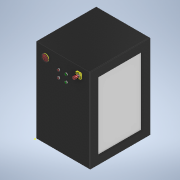
# Autodesk Inventor part: Tablero Maya
Saved by Autodesk Inventor 2020 (Build 240168000, 168)
## iProperties
Created: 2019-10-05
Part Number: Tablero Maya
Material: Genérico
Document SubType Name: Modeling
Designer: dasa1
Density: 1 g/cm^3
Appearance: Valor por defecto
Author: dasa1
Autodesk Inventor part; units mm, degrees
ref_plane "YZ Plane" through (0, 0, 0) normal (1, 0, 0) x (0, 1, 0)
ref_plane "XZ Plane" through (0, 0, 0) normal (0, 1, 0) x (-1, 0, 0)
ref_plane "XY Plane" through (0, 0, 0) normal (0, 0, 1) x (1, 0, 0)
sketch "Boceto1" plane through (0, 0, 0) normal (0, 1, 0) x (-1, 0, 0)
  line L0 (0, 0) -> (-530, 0)
  line L1 (-530, 0) -> (-530, -600)
  line L2 (-530, -600) -> (0, -600)
  line L3 (0, -600) -> (0, 0)
  dimension "d0" = 530
  dimension "d1" = 600
  constraints: 8 end point, 2 parallel, 1 horizontal, 1 perpendicular
  measures "d0" distance of L2.end L1.end
  measures "d1" distance of L1.end L0.end
extrude "Extrusión1" add sketch "Boceto1" along normal blind 840
sketch "Boceto2" plane through (530, 0, 0) normal (1, 0, 0) x (0, 0, -1)
  line L0 (0, 0) -> (0, 840) projected
  line L1 (0, 840) -> (10, 840)
  line L2 (10, 840) -> (10, 830)
  line L3 (10, 830) -> (0, 830)
  line L4 (0, 830) -> (0, 840)
  line L5 (10, 830) -> (590, 830)
  line L6 (590, 830) -> (590, 10)
  line L7 (590, 10) -> (10, 10)
  line L8 (10, 10) -> (10, 830)
  dimension "d4" = 10
  dimension "d5" = 10
  dimension "d6" = 580
  dimension "d7" = 820
  constraints: 16 end point, 4 parallel, 2 horizontal, 2 perpendicular
  measures "d4" distance of L2.end L3.end
  measures "d5" distance of L1.end L2.end
  measures "d6" distance of L6.end L7.end
  measures "d7" distance of L5.end L6.end
extrude "Extrusión2" cut sketch "Boceto2" against normal blind 520 contours L5 L6 L7 L8
sketch "Boceto3" plane through (0, 0, 0) normal (0, 0, 1) x (1, 0, 0)
  line L0 (530, 830) -> (10, 830) projected
  line L1 (10, 830) -> (520, 830) construction
  line L2 (520, 830) -> (520, 580) construction
  line L3 (520, 580) -> (10, 580) construction
  line L4 (10, 580) -> (10, 830) construction
  line L5 (265, 830) -> (265, 580) construction
  line L6 (265, 580) -> (265, 640)
  line L7 (265, 640) -> (290, 640) construction
  line L8 (265, 640) -> (240, 640) construction
  line L9 (290, 640) -> (302.5, 640) construction
  line L10 (240, 640) -> (227.5, 640) construction
  circle A0 centre (302.5, 640) radius 12.5
  circle A1 centre (227.5, 640) radius 12.5
  line L11 (227.5, 640) -> (227.5, 710) construction
  line L12 (302.5, 640) -> (302.5, 710) construction
  circle A2 centre (227.5, 710) radius 12.5
  circle A3 centre (302.5, 710) radius 12.5
  line L13 (10, 830) -> (10, 10) construction
  line L14 (10, 830) -> (10, 705) construction
  point P0 (0, 0)
  dimension "d10" = 510
  dimension "d11" = 250
  dimension "d12" = 255
  dimension "d13" = 0
  dimension "d14" = 60
  dimension "d15" = 25
  dimension "d16" = 25
  dimension "d17" = 12.5
  dimension "d18" = 12.5
  dimension "d19" = 70
  dimension "d20" = 70
  dimension "d21" = 25
  dimension "d22" = 25
  dimension "d23" = 125
  constraints: 26 end point, 4 coincident, 4 horizontal, 3 perpendicular, 2 centre point, 2 horizontal alignment, 2 parallel, 2 point on line, 2 vertical, 1 midpoint, 4 other
  measures "d10" distance of L2.end L3.end
  measures "d11" distance of L1.end L2.end
  measures "d12" distance between parallel lines of L5 L2
  measures "d13" distance from line of L5.start L0
  measures "d14" distance of L5.end L6.end
  measures "d15" distance of L6.end L7.end
  measures "d16" distance of L6.end L8.end
  measures "d17" distance of L7.end L9.end
  measures "d18" distance of L8.end L10.end
  measures "d19" distance of L11.start L11.end
  measures "d20" distance of L12.start L12.end
  measures "d21" diameter of A2
  measures "d22" diameter of A3
  measures "d23" distance of L0.end L14.end
extrude "Extrusión3" add sketch "Boceto3" along normal blind 10
sketch "Boceto4" plane through (302.5, 710, 10) normal (0, 0, 1) x (1, 0, 0)
  circle A0 centre (0, 0) radius 11.5
  circle A1 centre (-75, 0) radius 12.5 projected
  circle A2 centre (-75, 0) radius 11.5
  circle A3 centre (-75, 0) radius 12.5
  circle A4 centre (0, -70) radius 12.5 projected
  circle A5 centre (-75, 0) radius 12.5 projected
  circle A6 centre (-75, -70) radius 12.5 projected
  circle A7 centre (0, 0) radius 12.5 projected
  line L0 (-302.5, -710) -> (227.5, -710) projected
  line L1 (227.5, -710) -> (227.5, 130) projected
  line L2 (-302.5, 130) -> (227.5, 130) projected
  line L3 (-302.5, -710) -> (-302.5, 130) projected
  line L4 (-302.5, -710) -> (-302.5, 130) projected
  line L5 (0, 0) -> (-302.5, 0)
  line L6 (-302.5, 0) -> (-302.5, -710)
  line L7 (-302.5, -710) -> (0, -710)
  line L8 (0, -710) -> (0, 0)
  dimension "d26" = 23
  dimension "d27" = 23
  dimension "d29" = 75
  dimension "d30" = 710
  dimension "d31" = 302.5
  constraints: 8 end point, 3 centre point, 2 coincident, 2 parallel, 1 concentric, 1 horizontal, 1 perpendicular
  measures "d26" diameter of A0
  measures "d27" diameter of A2
  measures "d29" distance of A1.centre A0.centre
  measures "d30" distance of L7.end A0.centre
  measures "d31" distance of L0.start L7.end
extrude "Extrusión4" cut sketch "Boceto4" against normal blind 2 contours A0 L8 L5 | L5 L8 A0 | L5 A2 | A2 L5
fillet "Empalme1" radius 3 2 edges at (215, 640, 10) (290, 640, 10)
sketch "Boceto5" plane through (0, 0, 0) normal (0, 0, 1) x (1, 0, 0)
  circle A0 centre (302.5, 640) radius 12.5 projected
  circle A1 centre (227.5, 710) radius 12.5 projected
  circle A2 centre (227.5, 640) radius 12.5 projected
  circle A3 centre (302.5, 710) radius 12.5 projected
  line L0 (0, 0) -> (530, 0) projected
  line L1 (530, 0) -> (530, 840) projected
  line L2 (0, 840) -> (530, 840) projected
  line L3 (0, 0) -> (0, 840) projected
  line L4 (530, 830) -> (10, 830) construction
  line L5 (10, 830) -> (520, 830) construction
  line L6 (520, 830) -> (520, 630) construction
  line L7 (520, 630) -> (10, 630) construction
  line L8 (10, 630) -> (10, 830) construction
  line L9 (520, 630) -> (435, 630) construction
  line L10 (435, 630) -> (435, 770) construction
  line L11 (10, 630) -> (75, 630) construction
  line L12 (75, 630) -> (75, 770) construction
  line L13 (435, 770) -> (435, 795) construction
  line L14 (435, 795) -> (410, 795) construction
  line L15 (410, 795) -> (460, 795)
  line L16 (460, 795) -> (460, 745)
  line L17 (460, 745) -> (410, 745)
  line L18 (410, 745) -> (410, 795)
  dimension "d35" = 510
  dimension "d36" = 200
  dimension "d37" = 85
  dimension "d38" = 140
  dimension "d39" = 65
  dimension "d40" = 140
  dimension "d41" = 25
  dimension "d42" = 25
  dimension "d43" = 50
  dimension "d44" = 50
  constraints: 28 end point, 5 perpendicular, 4 parallel, 2 horizontal, 2 point on line, 1 vertical
  measures "d35" distance of L6.end L7.end
  measures "d36" distance of L5.end L6.end
  measures "d37" distance of L6.end L9.end
  measures "d38" distance of L9.end L10.end
  measures "d39" distance of L7.end L11.end
  measures "d40" distance of L11.end L12.end
  measures "d41" distance of L13.end L14.end
  measures "d42" distance of L10.end L13.end
  measures "d43" distance of L16.end L17.end
  measures "d44" distance of L15.end L16.end
extrude "Extrusión5" add sketch "Boceto5" along normal blind 15 contours L15 L16 L17 L18
sketch "Boceto7" plane through (0, 0, 15) normal (0, 0, 1) x (1, 0, 0)
  line L0 (410, 745) -> (460, 745) construction
  line L1 (460, 745) -> (460, 795) construction
  line L2 (460, 795) -> (410, 795) construction
  line L3 (410, 795) -> (410, 745) construction
  line L4 (460, 745) -> (410, 745) construction
  line L5 (410, 745) -> (435, 745) construction
  line L6 (435, 745) -> (435, 770) construction
  line L7 (435, 770) -> (410, 770) construction
  line L8 (410, 770) -> (410, 745) construction
  point P0 (0, 0)
  dimension "d53" = 25
  dimension "d54" = 25
  constraints: 8 end point, 2 parallel, 1 horizontal, 1 perpendicular
  measures "d53" distance of L7.end L6.end
  measures "d54" distance of L6.end L5.end
ref_plane "Plano de trabajo1" through (435, 770, 15) normal (-1, 0, 0) x (0, -1, 0)
sketch "Boceto8" plane through (435, 770, 15) normal (-1, 0, 0) x (0, -1, 0)
  line L0 (-25, 0) -> (25, 0) construction
  line L1 (0, 0) -> (0, 50)
  line L2 (0, 0) -> (50, 0) construction
  line L3 (0, 50) -> (-15, 50)
  line L4 (0, 50) -> (15, 50) construction
  line L5 (-15, 50) -> (-15, 40)
  line L6 (0, 0) -> (-10, 0)
  line L7 (-10, 0) -> (-15, 40)
  point P0 (770, -15)
  dimension "d55" = 50
  dimension "d56" = 90
  dimension "d57" = 15
  dimension "d58" = 180
  dimension "d59" = 10
  dimension "d60" = 10
  constraints: 14 end point, 3 horizontal, 2 equal length, 1 midpoint, 1 perpendicular, 1 point on line, 1 vertical
  measures "d55" distance of L1.start L1.end
  measures "d56" angle of L2 L1
  measures "d57" distance of L1.end L3.end
  measures "d58" angle of L3 L4
  measures "d59" distance of L3.end L5.end
  measures "d60" distance of L1.start L6.end
revolve "Revolución1" add sketch "Boceto8" angle 360 about axis through (435, 770, 15) along (0, 0, 1)
fillet "Empalme3" radius 5 1 edges at (435, 755, 65)
fillet "Empalme4" radius 5 1 edges at (435, 760, 15)
sketch "Boceto9" plane through (0, 0, 0) normal (0, 0, 1) x (1, 0, 0)
  line L0 (530, 830) -> (10, 830) construction
  line L1 (10, 830) -> (10, 10) construction
  line L2 (10, 830) -> (520, 830) construction
  line L3 (520, 830) -> (520, 630) construction
  line L4 (520, 630) -> (10, 630) construction
  line L5 (10, 630) -> (10, 830) construction
  line L6 (10, 630) -> (95, 630) construction
  line L7 (95, 630) -> (95, 750) construction
  line L8 (95, 750) -> (10, 750) construction
  line L9 (10, 750) -> (10, 630) construction
  line L10 (95, 750) -> (95, 785) construction
  circle A0 centre (95, 750) radius 35
  point P0 (0, 0)
  dimension "d64" = 510
  dimension "d65" = 200
  dimension "d66" = 85
  dimension "d67" = 120
  dimension "d68" = 35
  dimension "d69" = 70
  constraints: 18 end point, 4 parallel, 2 horizontal, 2 perpendicular, 1 centre point, 1 coincident, 1 vertical
  measures "d64" distance of L3.end L4.end
  measures "d65" distance of L2.end L3.end
  measures "d66" distance of L8.end L7.end
  measures "d67" distance of L7.end L6.end
  measures "d68" distance of L7.end L10.end
  measures "d69" diameter of A0
extrude "Extrusión7" add sketch "Boceto9" along normal blind 10
sketch "Boceto10" plane through (95, 750, 10) normal (0, 0, 1) x (1, 0, 0)
  circle A0 centre (0, 0) radius 30
  line L0 (0, 0) -> (0, 7) construction
  line L1 (0, 0) -> (-5, 0) construction
  line L2 (0, 0) -> (5, 0) construction
  line L3 (0, -30) -> (0, -29.5) construction
  line L4 (0, -29.5) -> (5.454356, -29.5) construction
  line L5 (0, -29.5) -> (-5.454356, -29.5) construction
  line L6 (0, -29.5) -> (-2.727178, -29.5) construction
  line L7 (0, -29.5) -> (2.727178, -29.5) construction
  line L8 (-5, 0) -> (0, 7)
  line L9 (0, 7) -> (5, 0)
  line L10 (2.727178, -29.5) -> (5, 0)
  line L11 (-5, 0) -> (-2.727178, -29.5)
  circle A1 centre (0, 0) radius 35
  circle A2 centre (0, 0) radius 29.625791
  point P0 (-95, -750)
  point P1 (2.727178, -29.5)
  dimension "d72" = 60
  dimension "d73" = 7
  dimension "d74" = 5
  dimension "d75" = 5
  dimension "d76" = 0.5
  constraints: 24 end point, 3 point on circle, 2 horizontal, 2 midpoint, 2 point on line, 2 vertical, 1 centre point, 1 coincident, 3 other
  measures "d72" diameter of A0
  measures "d73" distance of L0.start L0.end
  measures "d74" distance of L0.start L1.end
  measures "d75" distance of L0.start L2.end
  measures "d76" distance of L3.start L3.end
sketch "Boceto10 outline for Extrusión8" plane through (95, 750, 10) normal (0, 0, 1) x (1, 0, 0)
  line L0 (0, 7) -> (5, 0)
  line L1 (-5, 0) -> (0, 7)
  line L2 (-2.727178, -29.5) -> (-5, 0)
  arc A0 (2.727178, -29.5) -> (-2.727178, -29.5) centre (0, 0) ccw
  line L3 (5, 0) -> (2.727178, -29.5)
extrude "Extrusión8" cut sketch "Boceto10 outline for Extrusión8" against normal blind 9
sketch "Boceto11" plane through (95, 750, 10) normal (0, 0, 1) x (1, 0, 0)
  circle A0 centre (0, 0) radius 33.75
  point P0 (-95, -750)
  dimension "d79" = 67.5
  constraints: 1 centre point
  measures "d79" diameter of A0
extrude "Extrusión9" cut sketch "Boceto11" against normal blind 2
sketch "Boceto12" plane through (530, 0, 0) normal (1, 0, 0) x (0, 0, -1)
  line L0 (10, 830) -> (590, 830) construction
  line L1 (590, 830) -> (590, 10) construction
  line L2 (590, 10) -> (10, 10) construction
  line L3 (10, 10) -> (10, 830) construction
  line L4 (0, 0) -> (600, 0) construction
  line L5 (600, 0) -> (600, 840) construction
  line L6 (0, 840) -> (600, 840) construction
  line L7 (0, 0) -> (0, 840) construction
  line L8 (600, 0) -> (600, 840) construction
  line L9 (600, 840) -> (600, 720) construction
  line L10 (600, 0) -> (0, 0) construction
  line L11 (600, 0) -> (600, 120) construction
  line L12 (590, 830) -> (590, 10) projected
  line L13 (600, 120) -> (590, 120)
  line L14 (590, 120) -> (590, 200)
  line L15 (590, 200) -> (600, 200)
  line L16 (600, 200) -> (600, 120)
  line L17 (600, 720) -> (590, 720)
  line L18 (590, 720) -> (590, 640)
  line L19 (590, 640) -> (600, 640)
  line L20 (600, 640) -> (600, 720)
  dimension "d82" = 120
  dimension "d83" = 120
  dimension "d84" = 80
  dimension "d85" = 80
  constraints: 20 end point, 4 parallel, 4 point on line, 2 horizontal, 2 perpendicular
  measures "d82" distance of L5.end L9.end
  measures "d83" distance of L4.end L11.end
  measures "d84" distance of L13.end L14.end
  measures "d85" distance of L18.end L17.end
extrude "Extrusión10" add sketch "Boceto12" along normal blind 1
sketch "Boceto13" plane through (531, 0, 0) normal (1, 0, 0) x (0, 0, -1)
  line L0 (600, 0) -> (0, 0) projected
  line L1 (0, 0) -> (0, 840) projected
  line L2 (600, 840) -> (0, 840) projected
  line L3 (600, 0) -> (600, 840) projected
extrude "Extrusión11" add sketch "Boceto13" along normal blind 9
sketch "Boceto14" plane through (540, 0, 0) normal (1, 0, 0) x (0, 0, -1)
  line L0 (0, 0) -> (600, 0) construction
  line L1 (600, 0) -> (600, 840) construction
  line L2 (600, 840) -> (0, 840) construction
  line L3 (0, 840) -> (0, 0) construction
  line L4 (0, 840) -> (0, 0) construction
  line L5 (0, 840) -> (80, 840) construction
  line L6 (80, 840) -> (80, 760) construction
  line L7 (80, 760) -> (0, 760) construction
  line L8 (0, 760) -> (0, 840) construction
  line L9 (600, 0) -> (520, 0) construction
  line L10 (520, 0) -> (520, 80) construction
  line L11 (520, 80) -> (600, 80) construction
  line L12 (600, 80) -> (600, 0) construction
  line L13 (80, 760) -> (520, 760)
  line L14 (520, 760) -> (520, 80)
  line L15 (520, 80) -> (80, 80)
  line L16 (80, 80) -> (80, 760)
  dimension "d90" = 80
  dimension "d91" = 80
  dimension "d92" = 80
  dimension "d93" = 80
  constraints: 24 end point, 6 parallel, 3 horizontal, 3 perpendicular
  measures "d90" distance of L6.end L7.end
  measures "d91" distance of L5.end L6.end
  measures "d92" distance of L10.end L11.end
  measures "d93" distance of L9.end L10.end
extrude "Extrusión12" cut sketch "Boceto14" against normal blind 8
